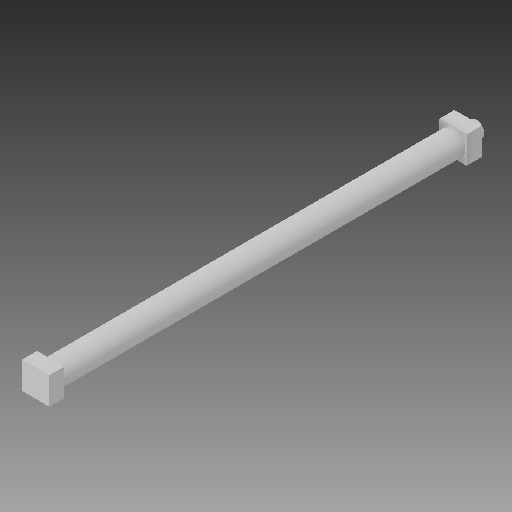
# Autodesk Inventor part: SC40-700
Saved by Autodesk Inventor 2019.4 (Build 234330000, 330)
## iProperties
Created: 2020-01-10
Part Number: SC40-700
Material: Generic
Document SubType Name: Modeling
Designer: Mark
Mass: 1321.84 g
Surface Area: 1235.65 cm^2
Volume: 1321.84 cm^3
Density: 1 g/cm^3
Appearance: Default
Author: Mark
Autodesk Inventor part; units mm, degrees
ref_plane "YZ Plane" through (0, 0, 0) normal (1, 0, 0) x (0, 1, 0)
ref_plane "XZ Plane" through (0, 0, 0) normal (0, 1, 0) x (-1, 0, 0)
ref_plane "XY Plane" through (0, 0, 0) normal (0, 0, 1) x (1, 0, 0)
sketch "Sketch1" plane through (0, 0, 0) normal (0, 0, 1) x (1, 0, 0)
  line L0 (-25, -25) -> (25, -25)
  line L1 (25, -25) -> (25, 25)
  line L2 (25, 25) -> (-25, 25)
  line L3 (-25, 25) -> (-25, -25)
  line L4 (-25, -25) -> (25, 25) construction
  line L5 (25, -25) -> (-25, 25) construction
  point P0 (0, 0)
  dimension "d0" = 50
  dimension "d1" = 50
  constraints: 12 end point, 2 midpoint, 2 parallel, 1 horizontal, 1 perpendicular
  measures "d0" distance of L2.end L1.end
  measures "d1" distance of L1.end L0.end
extrude "Extrusion1" add sketch "Sketch1" along normal blind 27.5
sketch "Sketch2" plane through (0, 0, 27.5) normal (0, 0, 1) x (1, 0, 0)
  circle A0 centre (0, 0) radius 22.5
  dimension "d4" = 45
  constraints: 1 centre point, 1 coincident
  measures "d4" diameter of A0
extrude "Extrusion2" add sketch "Sketch2" along normal blind 738
sketch "Sketch3" plane through (0, 0, 765.5) normal (0, 0, 1) x (1, 0, 0)
  line L0 (25, -25) -> (25, 25) projected
  line L1 (-25, -25) -> (25, -25)
  line L2 (25, -25) -> (25, 25)
  line L3 (25, 25) -> (-25, 25)
  line L4 (-25, 25) -> (-25, -25)
  line L5 (-25, -25) -> (25, 25) construction
  line L6 (25, -25) -> (-25, 25) construction
  point P0 (0, 0)
  constraints: 12 end point, 2 midpoint, 2 parallel, 1 horizontal, 1 perpendicular
extrude "Extrusion3" add sketch "Sketch3" along normal blind 27.5
sketch "Sketch4" plane through (0, 0, 0) normal (0, 0, -1) x (-1, 0, 0)
  circle A0 centre (0, 0) radius 15
  dimension "d9" = 30
  constraints: 1 centre point, 1 coincident
  measures "d9" diameter of A0
extrude "Extrusion4" add sketch "Sketch4" along normal blind 15
body "Solid1"
